# Autodesk Inventor part: XTAL_TXC_7A
Saved by Autodesk Inventor 2015 SP1 (Build 190203100, 203)
## iProperties
Created: 2015-06-25
Part Number: XTAL_TXC_7A
Material: Generic
Document SubType Name: Modeling
Designer: Patrick
Density: 1 g/cm^3
Appearance: 7A_SMD_XTAL, XTAL_TXC_7A
Author: Patrick
Autodesk Inventor part; units mm, degrees
ref_plane "YZ Plane" through (0, 0, 0) normal (1, 0, 0) x (0, 1, 0)
ref_plane "XZ Plane" through (0, 0, 0) normal (0, 1, 0) x (-1, 0, 0)
ref_plane "XY Plane" through (0, 0, 0) normal (0, 0, 1) x (1, 0, 0)
sketch "7A_SMD_XTAL, XTAL_TXC_7A_161" plane through (0, 0, 0) normal (0, 0, 1) x (1, 0, 0)
  line L0 (-2.7, -1.7) -> (-2.7, 1.7)
  line L1 (-2.7, 1.7) -> (2.7, 1.7)
  line L2 (2.7, 1.7) -> (2.7, -1.7)
  line L3 (2.7, -1.7) -> (-2.7, -1.7)
  constraints: 8 end point
extrude "Extrusion1" add sketch "7A_SMD_XTAL, XTAL_TXC_7A_161" along normal blind 1
body "Solid1"
